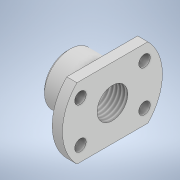
# Autodesk Inventor part: Втулка-12
Saved by Autodesk Inventor 2022 (Build 260153000, 153)
## iProperties
Created: 2021-12-03
Part Number: Втулка-12
Material: Типовые
Document SubType Name: Modeling
Designer: Украинцев
Density: 1 g/cm^3
Appearance: По умолчанию
Author: Украинцев
Autodesk Inventor part; units mm, degrees
ref_plane "YZ Plane" through (0, 0, 0) normal (1, 0, 0) x (0, 1, 0)
ref_plane "XZ Plane" through (0, 0, 0) normal (0, 1, 0) x (-1, 0, 0)
ref_plane "XY Plane" through (0, 0, 0) normal (0, 0, 1) x (1, 0, 0)
sketch "Эскиз1" plane through (0, 0, 0) normal (0, 1, 0) x (-1, 0, 0)
  line L0 (0, 0) -> (0, -39)
  line L1 (0, -39) -> (8, -39)
  line L2 (8, -39) -> (8, 0)
  line L3 (8, 0) -> (8, -19.75)
  line L4 (8, -19.75) -> (11, -19.75)
  line L5 (11, -19.75) -> (11, 0)
  line L6 (11, 0) -> (11, -20)
  line L7 (11, -20) -> (35, -20)
  line L8 (35, -20) -> (35, 0)
  line L9 (35, 0) -> (35, -12)
  line L10 (35, -12) -> (0, -12)
  line L11 (0, 0) -> (35, 0)
  line L12 (8, -19.75) -> (8, -20.75)
  line L13 (8, -20.75) -> (9, -20.75)
  circle A0 centre (9, -20.75) radius 1
  line L14 (11, -20) -> (9, -19.75)
  point P0 (9.2462, -19.7808)
  dimension "d0" = 39
  dimension "d1" = 8
  dimension "d2" = 19.75
  dimension "d3" = 3
  dimension "d4" = 20
  dimension "d6" = 12
  dimension "d27" = 1
  dimension "d28" = 1
  constraints: 30 end point, 7 perpendicular, 6 point on line, 2 point on circle, 2 vertical, 1 centre point, 1 coincident, 1 parallel
  measures "d0" distance of L0.start L0.end
  measures "d1" distance of L0.end L1.end
  measures "d2" distance of L2.end L3.end
  measures "d3" distance of L3.end L4.end
  measures "d4" distance of L6.end L5.end
  measures "d6" distance of L8.end L9.end
  measures "d27" distance of L3.end L12.end
  measures "d28" distance of L12.end L13.end
revolve "Вращение1" add sketch "Эскиз1" angle 360 about axis through (0, 0, 0) along (-1, 0, 0) contours L10 L2 L1 L0 | L10 L5 L4 L2 | L10 L8 L7 L6 L5
sketch "Эскиз2" plane through (0, 0, 0) normal (1, 0, 0) x (0, 0, -1)
  line L0 (25, -16) -> (-25, -16)
  line L1 (-25, -16) -> (-25, 16)
  line L2 (-25, 16) -> (25, 16)
  line L3 (25, 16) -> (25, -16)
  line L4 (25, -16) -> (-25, 16) construction
  line L5 (-25, -16) -> (25, 16) construction
  line L6 (0, 0) -> (0, -27.5)
  line L7 (0, -27.5) -> (39.6722, -27.5)
  line L8 (39.6722, -27.5) -> (-36.2697, -27.5)
  line L9 (0, 0) -> (0, 27.5)
  line L10 (0, 27.5) -> (-39.8646, 27.5)
  line L11 (-39.8646, 27.5) -> (34.879, 27.5)
  circle A0 centre (0, 0) radius 39
  point P0 (27.6541, 27.5)
  point P1 (-27.6541, 27.5)
  point P2 (-27.6541, -27.5)
  point P3 (27.6541, -27.5)
  dimension "d8" = 50
  dimension "d9" = 32
  dimension "d23" = 27.5
  dimension "d24" = 27.5
  constraints: 24 end point, 5 coincident, 3 perpendicular, 2 midpoint, 2 parallel, 2 point on line, 2 vertical, 1 centre point, 1 horizontal
  measures "d8" distance of L1.end L2.end
  measures "d9" distance of L0.end L1.end
  measures "d23" distance of L6.start L6.end
  measures "d24" distance of L6.start L9.end
hole "Отверстие1" at (0, -16, 25) at (0, 16, 25) at (0, 16, -25) at (0, -16, -25) direction (-1, 0, 0) diameter 9 end through all
chamfer "Фаска1" distance 2 angle 45 1 edges at (-35, 0, 20)
chamfer "Фаска2" distance 3 angle 45 1 edges at (-35, 0, 12)
extrude "Выдавливание1" cut sketch "Эскиз2" against normal through all contours L7 A0 L8 | L10 A0 L11
revolve "Вращение2" add sketch "Эскиз1" angle 360 about axis through (0, 0, 0) along (-1, 0, 0) contours L4 A0 L2 | L4 L6 L14 A0
thread "Резьба1" size "M24x3" class "6H" standard "ANSI Metric M Profile" full length
